Autodesk Fusion 360 part; units mm, degrees
(part 3 of 3)
sketch "Sketch22" plane through (0, 93.5, 0) normal (0, 1, 0) x (-1, 0, 0)
  circle A0 centre (-17.7, 4.5) radius 1.3
  circle A1 centre (-78, 12.2) radius 1.3
  circle A2 centre (-46.1, 25.7) radius 1.3
  circle A3 centre (-22.7, 25.7) radius 1.3
  line L0 (-61.05, 4.5) -> (-20.825, 4.5)
  arc A4 (-20.825, 4.5) -> (-14.575, 4.5) centre (-17.7, 4.5) ccw
  line L1 (-14.575, 4.5) -> (-6, 4.5)
  line L2 (-6, 4.5) -> (-6, 42.8)
  line L3 (-6, 42.8) -> (-30.75, 42.8)
  line L4 (-30.75, 42.8) -> (-30.75, 33.3)
  line L5 (-30.75, 33.3) -> (-98.4, 33.3)
  line L6 (-98.4, 33.3) -> (-98.4, 12.55)
  line L7 (-98.4, 12.55) -> (-93.55, 12.55)
  arc A5 (-92.05, 11.05) -> (-93.55, 12.55) centre (-93.55, 11.05) ccw
  line L8 (-92.05, 11.05) -> (-92.05, 4.5)
  line L9 (-92.05, 4.5) -> (-65.05, 4.5)
  line L10 (-65.05, 4.5) -> (-65.05, 10.55)
  arc A6 (-61.05, 10.55) -> (-65.05, 10.55) centre (-63.05, 10.55) ccw
  line L11 (-61.05, 10.55) -> (-61.05, 4.5)
  circle A7 centre (-22.7, 25.7) radius 3.125
  arc A8 (-20.825, 4.5) -> (-14.575, 4.5) centre (-17.7, 4.5) ccw
  circle A9 centre (-46.1, 25.7) radius 3.125
  circle A10 centre (-78, 12.2) radius 3.125
  line L12 (-96.4, 14.55) -> (-93.55, 14.55)
  arc A11 (-90.05, 11.05) -> (-93.55, 14.55) centre (-93.55, 11.05) ccw
  line L13 (-90.05, 11.05) -> (-90.05, 6.5)
  line L14 (-90.05, 6.5) -> (-67.05, 6.5)
  line L15 (-67.05, 6.5) -> (-67.05, 10.55)
  arc A12 (-59.05, 10.55) -> (-67.05, 10.55) centre (-63.05, 10.55) ccw
  line L16 (-59.05, 10.55) -> (-59.05, 6.5)
  line L17 (-59.05, 6.5) -> (-19.25, 6.5)
  arc A13 (-18.825, 4.5) -> (-18.8929, 5.0167) centre (-20.825, 4.5) ccw
  line L18 (-17.5, 6.5) -> (-8, 6.5)
  line L19 (-8, 6.5) -> (-8, 40.8)
  line L20 (-8, 40.8) -> (-28.75, 40.8)
  line L21 (-28.75, 40.8) -> (-28.75, 31.3)
  line L22 (-28.75, 31.3) -> (-96.4, 31.3)
  line L23 (-96.4, 31.3) -> (-96.4, 14.55)
  line L24 (-78.75, 15.2337) -> (-77.25, 15.2337)
  line L25 (-77.25, 15.2337) -> (-77.25, 31.3)
  line L26 (-77.25, 31.3) -> (-78.75, 31.3)
  line L27 (-78.75, 31.3) -> (-78.75, 15.2337)
  line L28 (-78.75, 9.1663) -> (-77.25, 9.1663)
  line L29 (-77.25, 9.1663) -> (-77.25, 6.5)
  line L30 (-77.25, 6.5) -> (-78.75, 6.5)
  line L31 (-78.75, 6.5) -> (-78.75, 9.1663)
  line L32 (-78.75, 20.3) -> (-96.4, 20.3)
  line L33 (-96.4, 18.8) -> (-78.75, 18.8)
  line L34 (-72.9, 31.3) -> (-72.9, 6.5)
  line L35 (-71.4, 31.3) -> (-71.4, 6.5)
  line L36 (-72.9, 21.75) -> (-75.75, 21.75)
  line L37 (-75.75, 21.75) -> (-75.75, 16.05)
  line L38 (-75.75, 16.05) -> (-72.9, 16.05)
  line L39 (-72.9, 16.9) -> (-74.9, 16.9)
  line L40 (-74.9, 16.9) -> (-74.9, 20.9)
  line L41 (-74.9, 20.9) -> (-72.9, 20.9)
  line L42 (-98.4, 33.3) -> (-98.4, 4.5) construction
  line L43 (-53.9, 31.3) -> (-53.9, 6.5)
  line L44 (-52.6, 31.3) -> (-52.6, 19.5)
  line L45 (-52.6, 19.5) -> (-46.7, 19.5)
  line L46 (-46.7, 19.5) -> (-46.7, 22.6331)
  line L47 (-46.7, 28.7669) -> (-46.7, 31.3)
  line L48 (-45.5, 31.3) -> (-45.5, 28.7669)
  line L49 (-45.5, 22.6331) -> (-45.5, 19.5)
  line L50 (-45.5, 19.5) -> (-30.5, 19.5)
  line L51 (-30.5, 19.5) -> (-30.5, 31.3)
  line L52 (-30.5, 18.3) -> (-45.5, 18.3)
  line L53 (-45.5, 18.3) -> (-45.5, 6.5)
  line L54 (-46.7, 6.5) -> (-46.7, 18.3)
  line L55 (-46.7, 18.3) -> (-52.6, 18.3)
  line L56 (-52.6, 18.3) -> (-52.6, 6.5)
  line L57 (-28.75, 31.3) -> (-28.75, 6.5)
  line L58 (-30.5, 18.3) -> (-30.5, 6.5)
  line L59 (-46.7, 19.5) -> (-46.7, 18.3) construction
  line L60 (-45.5, 19.5) -> (-46.7, 19.5) construction
  line L61 (-23.3, 28.7669) -> (-23.3, 40.8)
  line L62 (-22.1, 40.8) -> (-22.1, 28.7669)
  line L63 (-22.1, 34.7834) -> (-23.3, 34.7834) construction
  line L64 (-28.75, 19.5) -> (-8, 19.5)
  line L65 (-8, 19.5) -> (-8, 18.3)
  line L66 (-8, 18.3) -> (-28.75, 18.3)
  line L67 (-28.75, 18.3) -> (-28.75, 19.5)
  line L68 (-19.25, 6.5) -> (-17.5, 6.5)
  line L69 (-17.5, 6.5) -> (-17.5, 18.3)
  line L70 (-17.5, 18.3) -> (-19.25, 18.3)
  line L71 (-19.25, 18.3) -> (-19.25, 6.5)
  line L72 (-23.3, 22.6331) -> (-22.1, 22.6331)
  line L73 (-22.1, 22.6331) -> (-22.1, 19.5)
  line L74 (-22.1, 19.5) -> (-23.3, 19.5)
  line L75 (-23.3, 19.5) -> (-23.3, 22.6331)
  line L76 (-25.15, 17.075) -> (-19.5, 17.075)
  line L77 (-19.5, 17.075) -> (-19.5, 20.725)
  line L78 (-19.5, 20.725) -> (-25.15, 20.725)
  line L79 (-25.15, 20.725) -> (-25.15, 17.075)
  line L80 (-72.9, 16.05) -> (-71.4, 16.05)
  line L81 (-72.9, 21.75) -> (-71.4, 21.75)
  point P0 (-75.75, 18.9)
  point P1 (-98.4, 18.9)
  point P2 (-46.7, 18.9)
  point P3 (-46.1, 19.5)
  point P4 (-28.75, 18.9)
  point P5 (-18.375, 6.5)
  point P6 (-18.375, 18.3)
  point P7 (-25.15, 18.9)
  point P8 (-8, 18.9)
  dimension "d331" = 1.5
  dimension "d332" = 1.5
  dimension "d333" = 14.5
  dimension "d334" = 1.5
  dimension "d335" = 0.85
  dimension "d336" = 0.85
  dimension "d337" = 0.85
  dimension "d338" = 2
  dimension "d339" = 4
  dimension "d340" = 4.35
  dimension "d341" = 17.5
  dimension "d342" = 1.3
  dimension "d343" = 1.2
  dimension "d344" = 1.2
  dimension "d346" = 1.75
  dimension "d347" = 1.75
  dimension "d348" = 1.2
  dimension "d350" = 13.5
  dimension "d352" = 5.65
  dimension "d353" = 3.65
  constraint concentric A3 A7
  constraint equal A4 A7
  constraint concentric A2 A9
  constraint concentric A1 A10
  constraint equal A9 A10
  constraint equal A7 A9
  constraint concentric A5 A11
  constraint concentric A6 A12
  constraint coincident L0.end A4.start
  constraint tangent L15 A12
  constraint tangent L12 A11
  constraint tangent A11 L13
  constraint tangent A12 L16
  constraint tangent L17 A13
  constraint coincident A0 A13.end
  constraint horizontal L24
  constraint vertical L25
  constraint horizontal L26
  constraint vertical L27
  constraint coincident L22 L25.end
  constraint coincident A10 L24.start
  constraint coincident A10 L24.end
  constraint horizontal L28
  constraint vertical L29
  constraint horizontal L30
  constraint vertical L31
  constraint coincident L14 L29.end
  constraint coincident A10 L28.start
  constraint coincident A10 L28.end
  constraint equal L24 L28
  constraint coincident L27 L32.start
  constraint coincident L23 L32.end
  constraint perpendicular L23 L32
  constraint coincident L23 L33.start
  constraint coincident L27 L33.end
  constraint perpendicular L27 L33
  constraint coincident L22 L34.start
  constraint coincident L14 L34.end
  constraint perpendicular L14 L34
  constraint coincident L22 L35.start
  constraint coincident L14 L35.end
  constraint perpendicular L14 L35
  constraint coincident L34 L36.start
  constraint perpendicular L34 L36
  constraint perpendicular L36 L37
  constraint coincident L34 L38.end
  constraint perpendicular L34 L38
  constraint coincident L34 L39.start
  constraint perpendicular L34 L39
  constraint perpendicular L39 L40
  constraint coincident L34 L41.end
  constraint perpendicular L34 L41
  constraint coincident L5.end L6.start
  constraint perpendicular L9 L42
  constraint horizontal L8.end L42.end
  constraint midpoint L37 P0
  constraint midpoint L42 P1
  constraint horizontal P0 P1
  constraint coincident L22 L43.start
  constraint coincident L17 L43.end
  constraint perpendicular L17 L43
  constraint coincident L22 L44.start
  constraint perpendicular L22 L44
  constraint perpendicular L44 L45
  constraint coincident A9 L46.end
  constraint perpendicular L22 L46
  constraint coincident A9 L47.start
  constraint coincident L22 L47.end
  constraint perpendicular L22 L47
  constraint coincident L22 L48.start
  constraint coincident A9 L48.end
  constraint perpendicular L22 L48
  constraint coincident A9 L49.start
  constraint perpendicular L45 L49
  constraint perpendicular L46 L50
  constraint coincident L22 L51.end
  constraint perpendicular L22 L51
  constraint perpendicular L49 L52
  constraint coincident L17 L53.end
  constraint perpendicular L17 L53
  constraint coincident L17 L54.start
  constraint perpendicular L17 L54
  constraint perpendicular L54 L55
  constraint coincident L17 L56.end
  constraint perpendicular L17 L56
  constraint vertical L44.end L55.end
  constraint vertical L45.end L54.end
  constraint vertical L49.end L52.end
  constraint horizontal L45.end L49.end
  constraint horizontal L52.end L54.end
  constraint vertical L46.end L47.start
  constraint vertical L50.end L52.start
  constraint coincident L17 L57.end
  constraint perpendicular L17 L57
  constraint coincident L17 L58.end
  constraint perpendicular L17 L58
  constraint midpoint L59 P2
  constraint horizontal P1 P2
  constraint midpoint L60 P3
  constraint vertical A2.centre P3
  constraint vertical L48.end L49.start
  constraint coincident A7 L61.start
  constraint coincident L20 L61.end
  constraint perpendicular L20 L61
  constraint coincident L20 L62.start
  constraint coincident A7 L62.end
  constraint perpendicular L20 L62
  constraint midpoint L62 L63.start
  constraint midpoint L61 L63.end
  constraint perpendicular L61 L63
  constraint horizontal L64
  constraint vertical L65
  constraint horizontal L66
  constraint vertical L67
  constraint coincident L19 L65.end
  constraint coincident L57 L64.start
  constraint midpoint L67 P4
  constraint horizontal P1 P4
  constraint horizontal L50.end L64.start
  constraint horizontal L68
  constraint vertical L69
  constraint horizontal L70
  constraint vertical L71
  constraint coincident L66 L69.end
  constraint coincident L18.start L68.end
  constraint midpoint L68 P5
  constraint midpoint L66 P6
  constraint vertical P5 P6
  constraint horizontal L72
  constraint vertical L73
  constraint horizontal L74
  constraint vertical L75
  constraint coincident L64 L73.end
  constraint coincident A7 L72.start
  constraint vertical L62.end L72.end
  constraint vertical L61.start L72.start
  constraint horizontal L76
  constraint vertical L77
  constraint horizontal L78
  constraint vertical L79
  constraint midpoint L79 P7
  constraint midpoint L65 P8
  constraint horizontal P7 P8
  constraint coincident L35 L80.end
  constraint perpendicular L35 L80
  constraint coincident L35 L81.end
  constraint perpendicular L35 L81
  measures "d331" distance of L25 L27
  measures "d332" distance of L32 L33
  measures "d333" distance of L5 L33
  measures "d334" distance of L34 L35
  measures "d335" distance of L37 L40
  measures "d336" distance of L36 L41
  measures "d337" distance of L38 L39
  measures "d338" distance of L34 L40
  measures "d339" distance of L39 L41
  measures "d340" distance of L25 L34
  measures "d341" distance of L35 L43
  measures "d342" distance of L43 L44
  measures "d343" distance of L45 L55
  measures "d344" distance of L53 L54
  measures "d346" distance of L51 L57
  measures "d347" distance of L69 L71
  measures "d348" distance of L73 L75
  measures "d350" distance of L2 L77
  measures "d352" distance of L77 L79
  measures "d353" distance of L76 L78
extrude "Extrude53" cut sketch "Sketch22" against normal blind 10 contours A7 L19 L20 L62 L64 L73 L77 L78 | A7 L20 L21 L57 L61 L64 L75 L78 L79 | L18 L19 L66 L69 | L17 L57 L66 L71 L76 L77 L79 | A9 L22 L48 L49 L50 L51 | A9 L22 L44 L45 L46 L47 | L17 L52 L53 L58 | L14 L15 A12 L16 L17 L22 L35 L43 | L17 L54 L55 L56 | A10 L14 L22 L25 L29 L34 L36 L37 L38 | L22 L23 L27 L32 | L34 L39 L40 L41 | A10 L12 A11 L13 L14 L23 L27 L31 L33
extrude "Extrude54" add sketch "Sketch22" along normal blind 1 contours L64 L73 L77 L78 | L64 L73 L74 L75 L78 | L64 L75 L78 L79 | L64 L66 L74 L77 L79 | L66 L76 L77 L79 | L34 L35 L80 L81 | L34 L36 L37 L38 L39 L40 L41
fillet "Fillet3" radius 3.5 1 edges at (38.2, 4.15, 47.8)
fillet "Fillet4" radius 1.5 1 edges at (40.2, 3.3, 45.8)
sketch "Sketch23" plane through (111.4, 0, 0) normal (1, 0, 0) x (0, 0, -1)
  line L0 (0, 34.9) -> (-19.1, 34.9)
  line L1 (-19.1, 34.9) -> (-19.1, 71.5)
  line L2 (-19.1, 71.5) -> (-33.3, 71.5)
  line L3 (-33.3, 71.5) -> (-33.3, 0)
  line L4 (-33.3, 0) -> (0, 0)
  line L5 (0, 0) -> (0, 34.9)
  line L6 (-14.6, 34.9) -> (-14.6, 15.9)
  line L7 (0, 0) -> (-14.6, 15.9)
  dimension "d363" = 4.5
  dimension "d364" = 19
  constraint coincident L0 L6.start
  constraint perpendicular L0 L6
  constraint coincident L4.end L5.start
  measures "d363" distance of L0.end L6.start
  measures "d364" distance of L6.start L6.end
extrude "Extrude55" cut sketch "Sketch23" against normal up to surface (1.75 mm away) contours L0 L5 L6 L7
equation "d31 = 4.25 mm + 4 mm"
equation "d61 = 29.9 mm - 1.165 mm"
equation "d94 = 11.5 mm - ( 5.05 / 2 ) * 1 mm"
equation "d107 = 11.5 mm - ( 5.05 / 2 ) * 1 mm"
equation "d120 = 11.5 mm - ( 5.05 / 2 ) * 1 mm"
equation "d133 = 11.5 mm - ( 5.05 / 2 ) * 1 mm"
equation "d150 = 22.5 mm + ( 0.7 / 2 ) * 1 mm"
equation "d165 = 19.1 mm + ( 2.6 / 2 ) * 1 mm"
equation "d166 = 6.4 mm + ( 2.6 / 2 ) * 1 mm"
equation "d169 = 6.3 mm + ( 2.6 / 2 ) * 1 mm"
equation "d170 = 38.8 mm + ( 2.6 / 2 ) * 1 mm"
equation "d171 = 15.4 mm + ( 2.6 / 2 ) * 1 mm"
equation "d173 = 10.5 mm + ( 2.5 / 2 ) * 1 mm"
equation "d185 = 21.5 mm + ( 2.65 / 2 ) * 1 mm"
equation "d186 = 27.35 mm + ( 2.65 / 2 ) * 1 mm"
equation "d199 = d198"
equation "d203 = d202"
equation "d204 = d202"
equation "d205 = d202"
equation "d206 = d202"
equation "d212 = d211"
equation "d213 = d212"
equation "d216 = d214"
equation "d217 = d213"
equation "d222 = d221"
equation "d223 = d221"
equation "d224 = d221"
equation "d226 = d221"
equation "d227 = d221"
equation "d228 = d221"
equation "d229 = d221"
equation "d230 = d221"
equation "d231 = d221"
equation "d233 = d221"
equation "d243 = d240"
equation "d246 = d237"
equation "d256 = d255"
equation "d257 = d256"
equation "d258 = d256"
equation "d260 = d255"
equation "d261 = d247"
equation "d279 = 10.5 mm + ( 2.4 / 2 ) * 1 mm"
equation "d294 = d293"
equation "d297 = d296"
equation "d298 = d297"
equation "d299 = d298"
equation "d300 = d296"
equation "d301 = d299"
equation "d302 = d300"
equation "d303 = d300"
equation "d305 = d304"
equation "d307 = d306"
equation "d309 = d294"
equation "d311 = d309"
equation "d332 = d331"
equation "d334 = d331"
equation "d336 = d335"
equation "d337 = d336"
equation "d344 = d343"
equation "d347 = d346"
equation "d348 = d344"
